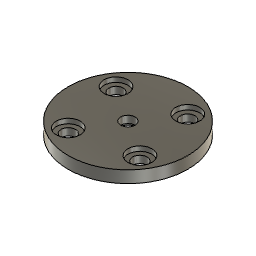
_Motorised arm cap _ motor attachment.abfe61bb-9a0f-4074-8c70-eef68518f80a (Autodesk Fusion 360 design; units mm, degrees)
Autodesk Fusion 360 part; units mm, degrees
sketch "Sketch1" plane through (0, 0, 0) normal (0, 0, 1) x (1, 0, 0)
  circle A0 centre (0, 0) radius 25
  dimension "d1" = 50
  constraint coincident A0.centre origin
  measures "d1" diameter of A0
extrude "Extrude1" add sketch "Sketch1" along normal blind 5
sketch "Sketch2" plane through (0, 0, 5) normal (0, 0, 1) x (-1, 0, 0)
  circle A0 centre (0, 0) radius 25
  circle A1 centre (15, -10) radius 3
  circle A2 centre (-10, -15) radius 3
  circle A3 centre (-15, 10) radius 3
  circle A4 centre (10, 15) radius 3
  dimension "d4" = 6
  dimension "d5" = 6
  dimension "d6" = 6
  dimension "d7" = 6
  measures "d4" diameter of A1
  measures "d5" diameter of A2
  measures "d6" diameter of A3
  measures "d7" diameter of A4
extrude "Extrude2" cut sketch "Sketch2" against normal blind 5 contours A1 | A2 | A3 | A4
sketch "Sketch3" plane through (0, 0, 5) normal (0, 0, 1) x (-1, 0, 0)
  circle A0 centre (-10, -15) radius 3
  circle A1 centre (-15, 10) radius 3
  circle A2 centre (15, -10) radius 3
  circle A3 centre (10, 15) radius 3
  circle A4 centre (0, 0) radius 25
  circle A5 centre (15, -10) radius 5
  circle A6 centre (-10, -15) radius 5
  circle A7 centre (-15, 10) radius 5
  circle A8 centre (10, 15) radius 5
  dimension "d10" = 10
  dimension "d11" = 10
  dimension "d12" = 10
  dimension "d13" = 10
  constraint concentric A2 A5
  constraint concentric A0 A6
  constraint concentric A1 A7
  constraint concentric A3 A8
  measures "d10" diameter of A5
  measures "d11" diameter of A6
  measures "d12" diameter of A7
  measures "d13" diameter of A8
extrude "Extrude3" cut sketch "Sketch3" against normal blind 2 contours A5 | A6 | A7 | A8
sketch "Sketch4" plane through (0, 0, 5) normal (0, 0, 1) x (-1, 0, 0)
  circle A0 centre (-10, -15) radius 5
  circle A1 centre (-15, 10) radius 5
  circle A2 centre (15, -10) radius 5
  circle A3 centre (10, 15) radius 5
  circle A4 centre (0, 0) radius 25
  circle A5 centre (0, 0) radius 3
  dimension "d16" = 6
  constraint coincident A4.centre A5.centre
  measures "d16" diameter of A5
extrude "Extrude4" cut sketch "Sketch4" against normal blind 21 contours A5
sketch "Sketch5" plane through (0, 0, 0) normal (0, 0, 1) x (1, 0, 0)
  circle A0 centre (0, 0) radius 5
  dimension "d19" = 10
  constraint coincident A0.centre origin
  measures "d19" diameter of A0
extrude "Extrude5" cut sketch "Sketch5" along normal blind 2
